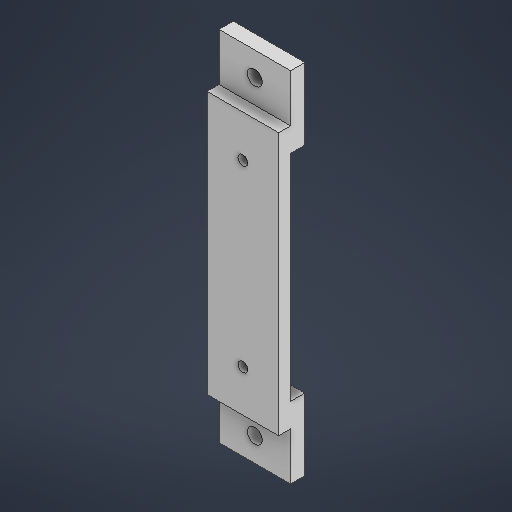
# Autodesk Inventor part: DepthCAM
Saved by Autodesk Inventor 2026.2 (Build 302298000, 298)
## iProperties
Created: 2026-01-08
Part Number: DepthCAM
Material: Generisch
Document SubType Name: Modeling
Designer: Alex
Density: 1 g/cm^3
Appearance: Vorgabe
Author: Alex
Autodesk Inventor part; units mm, degrees
ref_plane "YZ Plane" through (0, 0, 0) normal (1, 0, 0) x (0, 1, 0)
ref_plane "XZ Plane" through (0, 0, 0) normal (0, 1, 0) x (-1, 0, 0)
ref_plane "XY Plane" through (0, 0, 0) normal (0, 0, 1) x (1, 0, 0)
sketch "Skizze1" plane through (0, 0, 0) normal (0, 1, 0) x (-1, 0, 0)
  line L0 (-15, 50) -> (15, 50)
  line L1 (15, 50) -> (15, -50)
  line L2 (15, -50) -> (-15, -50)
  line L3 (-15, -50) -> (-15, 50)
  line L4 (-15, 50) -> (15, -50) construction
  line L5 (15, 50) -> (-15, -50) construction
  point P0 (0, 0)
  dimension "d0" = 30
  dimension "d1" = 100
  constraints: 12 end point, 2 midpoint, 2 parallel, 1 horizontal, 1 perpendicular
  measures "d0" distance of L1.end L2.end
  measures "d1" distance of L0.end L1.end
extrude "Extrusion1" add sketch "Skizze1" along normal blind 5
sketch "Skizze2" plane through (0, 5, 0) normal (0, 1, 0) x (1, 0, 0)
  line L0 (15, 50) -> (-15, 50) projected
  line L1 (-15, 50) -> (-15, -50) projected
  line L2 (-15, -50) -> (15, -50) projected
  line L3 (15, -50) -> (15, 50) projected
  line L4 (-15, -50) -> (15, -50) projected
  line L5 (0, -37.5) -> (0, 37.5)
  circle A0 centre (0, -37.5) radius 2.05
  circle A1 centre (0, 37.5) radius 2.05
  point P0 (0, 0)
  dimension "d22" = 75
  dimension "d23" = 4.1
  dimension "d24" = 4.1
  constraints: 2 centre point, 2 coincident, 2 end point
  measures "d22" distance of L5.start L5.end
  measures "d23" diameter of A0
  measures "d24" diameter of A1
sketch "Skizze3" plane through (0, 5, 0) normal (0, 1, 0) x (1, 0, 0)
  line L0 (-15, -50) -> (15, -50) projected
  line L1 (-15, -50) -> (0, -50)
  line L2 (0, -37.5) -> (0, 37.5)
  circle A0 centre (0, -37.5) radius 2.05
  circle A1 centre (0, 37.5) radius 2.05
  line L3 (15, -50) -> (15, 50) projected
  line L4 (-15, -50) -> (15, -50)
  line L5 (15, -50) -> (15, -45)
  line L6 (15, -45) -> (-15, -45)
  line L7 (-15, -45) -> (-15, -50)
  line L8 (-15, 50) -> (15, 50)
  line L9 (15, 50) -> (15, 45)
  line L10 (15, 45) -> (-15, 45)
  line L11 (-15, 45) -> (-15, 50)
  point P0 (0, 0)
  dimension "d4" = 15
  dimension "d5" = 12.5
  dimension "d6" = 75
  dimension "d7" = 4.1
  dimension "d8" = 4.1
  dimension "d9" = 5
  dimension "d10" = 5
  constraints: 20 end point, 4 parallel, 3 point on line, 2 centre point, 2 coincident, 2 horizontal, 2 perpendicular, 1 midpoint
  measures "d4" distance of L0.start L1.end
  measures "d5" distance of L1.end L2.start
  measures "d6" distance of L2.start L2.end
  measures "d7" diameter of A0
  measures "d8" diameter of A1
  measures "d9" distance of L5.end L4.end
  measures "d10" distance of L8.end L9.end
extrude "Extrusion2" add sketch "Skizze3" along normal blind 6 contours L7 L6 L3 L0 | L10 L11 L8 L3
sketch "Skizze4" plane through (-15, 0, 50) normal (0, 0, 1) x (1, 0, 0)
  line L0 (0, 0) -> (30, 0) projected
  line L1 (30, 0) -> (30, 11) projected
  line L2 (0, 11) -> (30, 11) projected
  line L3 (0, 0) -> (0, 11) projected
  line L4 (0, 5) -> (30, 5) projected
  point P0 (15, 0)
extrude "Extrusion3" add sketch "Skizze4" along normal blind 25 contours L3 L2 L1 L4
sketch "Skizze5" plane through (15, 0, -50) normal (0, 0, -1) x (-1, 0, 0)
  line L0 (0, 0) -> (30, 0) projected
  line L1 (30, 0) -> (30, 11) projected
  line L2 (0, 11) -> (30, 11) projected
  line L3 (0, 0) -> (0, 11) projected
  line L4 (0, 5) -> (30, 5) projected
  point P0 (15, 0)
extrude "Extrusion4" add sketch "Skizze5" along normal blind 25 contours L3 L2 L1 L4
sketch "Skizze6" plane through (15, 0, -50) normal (0, 0, -1) x (-1, 0, 0)
  line L0 (0, 5) -> (30, 5) projected
  line L1 (0, 0) -> (30, 0) projected
  line L2 (30, 5) -> (0, 5) projected
  line L3 (0, 0) -> (0, 5) projected
  line L4 (0, 0) -> (30, 0) projected
  line L5 (30, 0) -> (30, 5) projected
  point P0 (15, 0)
extrude "Extrusion5" add sketch "Skizze6" along normal blind 5
sketch "Skizze7" plane through (-15, 0, 50) normal (0, 0, 1) x (1, 0, 0)
  line L0 (30, 5) -> (0, 5) projected
  line L1 (0, 0) -> (0, 5) projected
  line L2 (0, 0) -> (30, 0) projected
  line L3 (30, 0) -> (30, 5) projected
  point P0 (15, 0)
extrude "Extrusion6" add sketch "Skizze7" along normal blind 5
extrude "Extrusion7" cut sketch "Skizze2" against normal blind 5 contours A1 | A0
sketch "Skizze8" plane through (0, 11, 0) normal (0, 1, 0) x (1, 0, 0)
  line L0 (15, -45) -> (15, -75) projected
  line L1 (15, -45) -> (-15, -45) projected
  line L2 (-15, -45) -> (-15, -75) projected
  line L3 (15, -75) -> (-15, -75) projected
  line L4 (0, -75) -> (0, -65)
  circle A0 centre (0, -65) radius 3.1
  line L5 (-15, 45) -> (-15, 75) projected
  line L6 (-15, 45) -> (15, 45) projected
  line L7 (15, 45) -> (15, 75) projected
  line L8 (-15, 75) -> (15, 75) projected
  line L9 (0, 75) -> (0, 65)
  circle A1 centre (0, 65) radius 3.1
  point P0 (0, 0)
  dimension "d27" = 10
  dimension "d28" = 6.2
  dimension "d29" = 10
  dimension "d30" = 6.2
  constraints: 4 end point, 2 centre point, 2 coincident, 2 midpoint, 2 vertical
  measures "d27" distance of L4.start L4.end
  measures "d28" diameter of A0
  measures "d29" distance of L9.start L9.end
  measures "d30" diameter of A1
extrude "Extrusion8" cut sketch "Skizze8" against normal blind 7 contours A0 | A1
